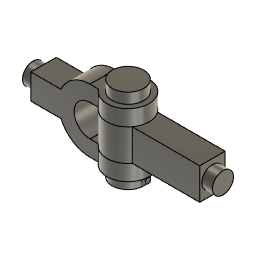
Sketch30_Final v1 (Autodesk Fusion 360 design; units mm, degrees)
Autodesk Fusion 360 part; units mm, degrees
sketch "Sketch1" plane through (0, 0, 0) normal (0, 1, 0) x (1, 0, 0)
  circle A0 centre (0, 0) radius 50
  line L0 (200, 0) -> (200, -30)
  line L1 (200, -30) -> (40, -30)
  line L2 (200, 0) -> (200, 30)
  line L3 (200, 30) -> (40, 30)
  line L4 (225, 0) -> (225, 25)
  line L5 (225, 25) -> (200, 25)
  line L6 (225, 0) -> (225, -25)
  line L7 (225, -25) -> (200, -25)
  circle A1 centre (0, 0) radius 25
  line L8 (200, 0) -> (225, 0)
  dimension "d6" = 100
  dimension "d7" = 200
  dimension "d8" = 30
  dimension "d9" = 25
  dimension "d10" = 25
  dimension "d11" = 25
  dimension "d12" = 50
  constraint coincident A0.centre A1.centre
  constraint coincident A0 L1.end
  constraint perpendicular L0 L1
  constraint coincident A0 L3.end
  constraint perpendicular L2 L3
  constraint coincident L2 L5.end
  constraint perpendicular L2 L5
  constraint coincident L0 L7.end
  constraint perpendicular L0 L7
  constraint perpendicular L6 L8
  measures "d6" diameter of A0
  measures "d7" distance of A0.centre L0.start
  measures "d8" distance of L0.start L0.end
  measures "d9" distance of L0.start L4.start
  measures "d10" distance of L4.start L4.end
  measures "d11" distance of L4.start L6.end
  measures "d12" diameter of A1
sketch "Sketch3" plane through (0, 0, 0) normal (0, 1, 0) x (1, 0, 0)
  line L0 (0, 0) -> (-25, 0)
  line L1 (0, 0) -> (-50, 0)
  line L2 (0, 0) -> (0, -175)
  line L3 (0, -175) -> (-60, -175)
  line L4 (-60, -175) -> (-60, -137.5)
  line L5 (-60, -137.5) -> (0, -137.5)
  line L6 (0, -137.5) -> (-37.5, -137.5)
  line L7 (0, 0) -> (0, -100)
  line L8 (0, -100) -> (-135, -100)
  line L9 (-60, -175) -> (-60, -100)
  arc A0 (-135, -100) -> (-60, -175) centre (-60, -100) ccw
  arc A1 (-97.5, -100) -> (-60, -137.5) centre (-60, -100) ccw
  arc A2 (-60, -62.5) -> (-97.5, -100) centre (-60, -100) ccw
  arc A3 (-60, -25) -> (-135, -100) centre (-60, -100) ccw
  line L10 (-60, -62.5) -> (0, -62.5)
  line L11 (0, -25) -> (-60, -25)
  line L12 (0, -100) -> (-200, -100)
  line L13 (-200, -100) -> (-200, -130)
  line L14 (-200, -130) -> (-128.7386, -130)
  line L15 (-200, -70) -> (-128.7386, -70)
  line L16 (-200, -100) -> (-200, -70)
  line L17 (-200, -100) -> (-225, -100)
  line L18 (-225, -100) -> (-225, -125)
  line L19 (-225, -125) -> (-200, -125)
  dimension "d18" = 25
  dimension "d19" = 50
  dimension "d21" = 175
  dimension "d22" = 60
  dimension "d23" = 37.5
  dimension "d24" = 37.5
  dimension "d25" = 100
  dimension "d28" = 200
  dimension "d29" = 25
  dimension "d30" = 25
  constraint coincident L0.start L1.start
  constraint horizontal L0
  constraint parallel L0 L1
  constraint perpendicular L1 L2
  constraint perpendicular L2 L3
  constraint perpendicular L3 L4
  constraint coincident L2 L5.end
  constraint perpendicular L2 L5
  constraint perpendicular L2 L6
  constraint perpendicular L0 L7
  constraint perpendicular L7 L8
  constraint coincident L8 L9.end
  constraint perpendicular L8 L9
  constraint coincident L9.end A0.centre
  constraint concentric A0 A1
  constraint coincident L8 A1.start
  constraint symmetric L2.end L8 L11.start
  constraint symmetric L3.end L8 A3.start
  constraint symmetric L4.end L8 A2.start
  constraint symmetric L5.end L8 L10.end
  constraint symmetric L8 A0 A3
  constraint symmetric L8 A1.start A2.end
  constraint symmetric L8 A1 A2
  constraint coincident A0 L14.end
  constraint perpendicular L12 L13
  constraint symmetric L14.end L12 L15.end
  constraint symmetric L13.start L12 L16.start
  constraint symmetric L12 L13.end L15.start
  constraint perpendicular L13 L17
  constraint perpendicular L17 L18
  constraint coincident L13 L19.end
  constraint perpendicular L13 L19
  measures "d18" distance of L0.start L0.end
  measures "d19" distance of L0.start L1.end
  measures "d21" distance of L0.start L2.end
  measures "d22" distance of L2.end L3.end
  measures "d23" distance of L3.end L4.end
  measures "d24" distance of L5.end L6.end
  measures "d25" distance of L0.start L7.end
  measures "d28" distance of L7.end L12.end
  measures "d29" distance of L12.end L17.end
  measures "d30" distance of L17.end L18.end
extrude "Extrude2" add sketch "Sketch3" along normal mid plane 60 contours L2 L7 L8 A2 A3 L10 L11 L12 | A3 L12 L15 L16 | L2 L3 L4 L5 L6 L9 | L4 L8 L9 A0 A1 L12 | A0 L12 L13 L14 makes body 1
revolve "Revolve2" add sketch "Sketch3" angle 360 about axis through (0, 0, 100) along (-1, 0, 0) contours L13 L17 L18 L19 bodies 1
ref_plane "WorkPlane1" through (0, 0, 25) normal (0, 0, 1) x (1, 0, 0)
sketch "Sketch4" plane through (0, 0, 25) normal (0, 0, 1) x (1, 0, 0)
  circle A0 centre (0, 0) radius 25
  circle A1 centre (0, 0) radius 50
  dimension "d35" = 50
  dimension "d36" = 100
  constraint coincident A0.centre A1.centre
  measures "d35" diameter of A0
  measures "d36" diameter of A1
extrude "Extrude3" add sketch "Sketch4" along normal blind 37.5 bodies 1
extrude "Extrude4" cut sketch "Sketch4" along normal blind 37.5 contours A0 bodies 1
ref_plane "WorkPlane3" through (-5, 0, 137.5) normal (0, 0, 1) x (1, 0, 0)
sketch "Sketch5" plane through (-5, 0, 137.5) normal (0, 0, 1) x (1, 0, 0)
  circle A0 centre (5, 0) radius 25
  circle A1 centre (5, 0) radius 50
  dimension "d43" = 50
  dimension "d44" = 100
  constraint concentric A0 A1
  measures "d43" diameter of A0
  measures "d44" diameter of A1
extrude "Extrude5" add sketch "Sketch5" along normal blind 37.5 bodies 1
extrude "Extrude6" cut sketch "Sketch5" along normal blind 37.5 contours A0 bodies 1
copy_body "Body->Comp2" bodies 1 removing the originals makes body 2 in component "Fork"
sketch "Sketch7" plane through (0, 0, 0) normal (0, 0, 1) x (1, 0, 0)
  circle A0 centre (0, 0) radius 25
  circle A1 centre (0, 0) radius 37.5
  dimension "d49" = 50
  dimension "d50" = 75
  constraint coincident A0.centre A1.centre
  constraint concentric A0 A1
  measures "d49" diameter of A0
  measures "d50" diameter of A1
extrude "Extrude7" add sketch "Sketch7" along normal mid plane 25 separate body makes body 3
copy_body "Body->Comp3" bodies 3 removing the originals makes body 4 in component "Collar"
hole "Hole1" at (37.5, 0, 2.7878) direction (-1, 0, 0) diameter 12.5 depth 80 tip angle 118 bodies 4 in component "Collar"
sketch "Sketch8" plane through (0, 0, 0) normal (0, 1, 0) x (1, 0, 0)
  line L0 (0, 0) -> (0, -6.25)
  line L1 (0, -6.25) -> (50, -6.25)
  line L2 (50, -6.25) -> (50, 0)
  line L3 (50, 0) -> (0, 0)
  line L4 (0, -6.25) -> (-50, -6.25)
  line L5 (-50, 0) -> (0, 0)
  line L6 (-50, -6.25) -> (-50, 0)
  dimension "d56" = 6.25
  dimension "d57" = 50
  constraint coincident L0.start L3.end
  constraint vertical L0
  constraint perpendicular L0 L1
  constraint perpendicular L1 L2
  constraint perpendicular L0 L3
  constraint symmetric L1.start L0 L4.start
  constraint symmetric L0 L1.end L4.end
  constraint symmetric L0 L2.end L5.start
  constraint symmetric L0 L3.end L5.end
  measures "d56" distance of L0.start L0.end
  measures "d57" distance of L0.end L1.end
revolve "Revolve3" add sketch "Sketch8" angle 360 about axis through (50, 0, 0) along (-1, 0, 0) separate body makes body 5
copy_body "Body->Comp4" bodies 5 removing the originals makes body 6 in component "Pin"
sketch "Sketch9" plane through (0, 0, 0) normal (0, 1, 0) x (1, 0, 0)
  line L0 (0, 0) -> (0, -200)
  line L1 (0, -200) -> (37.5, -200)
  line L2 (37.5, -200) -> (37.5, -175)
  line L3 (37.5, -175) -> (25, -175)
  line L4 (25, -175) -> (25, 0)
  line L5 (25, 0) -> (0, 0)
  dimension "d59" = 200
  dimension "d60" = 37.5
  dimension "d61" = 25
  constraint coincident L0.start L5.end
  constraint vertical L0
  constraint perpendicular L0 L1
  constraint perpendicular L1 L2
  constraint perpendicular L2 L3
  constraint perpendicular L3 L4
  constraint perpendicular L0 L5
  measures "d59" distance of L0.start L0.end
  measures "d60" distance of L0.end L1.end
  measures "d61" distance of L1.end L2.end
revolve "Revolve4" add sketch "Sketch9" angle 360 about axis through (0, 0, 0) along (0, 0, 1) separate body makes body 7
copy_body "Body->Comp5" bodies 7 removing the originals makes body 8 in component "TaperPin"
hole "Hole1'" at (25, 0, 12.5) direction (-1, 0, 0) diameter 12.5 depth 80 tip angle 118 bodies 8 in component "TaperPin"
extrude "Extrude8" add sketch "Sketch1" along normal mid plane 75 separate body contours A0 | A0 L0 L1 L2 L3 makes body 9
revolve "Revolve5" add sketch "Sketch1" angle 360 about axis through (1.75, 0, 0) along (1, 0, 0) contours L0 L6 L7 L8 bodies 9
copy_body "Body->Comp6" bodies 9 removing the originals makes body 10 in component "Eye"
component "Fork" placed x (-1, 0, 0) y (0, -1, 0) z (0, 0, 1) at (89.6893, 230.5645, 128.3752)
component "Collar" placed x (1, 0, 0) y (0, 1, 0) z (0, 0, 1) at (89.6893, 230.5645, 140.8752)
component "Pin" placed x (-1, 0, 0) y (0, -1, 0) z (0, 0, 1) at (92.1921, 230.5645, 143.663)
component "TaperPin" placed x (-1, 0, 0) y (0, -1, 0) z (0, 0, 1) at (89.6893, 230.5645, 128.3752)
component "Eye" placed x (-1, 0, 0) y (0, 0, 1) z (0, 1, 0) at (89.6893, 230.5645, 228.3752)
named bodies: "Fork", "Collar", "Pin", "TaperPin", "Eye"
